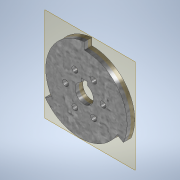
# Autodesk Inventor part: Weapon
Saved by Autodesk Inventor 2022 (Build 260153000, 153)
## iProperties
Created: 2022-08-11
Part Number: Weapon
Material: Steel
Document SubType Name: Sheet Metal
Designer: Nick
Density: 7.85 g/cm^3
Appearance: Steel Galvanized
Mass: 169.361 g
Surface Area: 86.0381 cm^2
Volume: 21.5746 cm^3
Flat Pattern Width: 6.80954 cm
Flat Pattern Length: 7.10597 cm
Flat Pattern Area: 48.3884 cm^2
Sheet Metal Rule: Default
Sheet Metal Width: 2.681 in
Sheet Metal Length: 2.798 in
Sheet Metal Area: 7.500 in^2
Author: Nick
Autodesk Inventor part; units mm, degrees
ref_plane "YZ Plane" through (0, 0, 0) normal (1, 0, 0) x (0, 1, 0)
ref_plane "XZ Plane" through (0, 0, 0) normal (0, 1, 0) x (-1, 0, 0)
ref_plane "XY Plane" through (0, 0, 0) normal (0, 0, 1) x (1, 0, 0)
sketch "Sketch1" plane through (0, 0, 0) normal (0, 0, 1) x (1, 0, 0)
  circle A0 centre (0, 0) radius 37.5 construction
  circle A1 centre (0, 0) radius 31.5
  line L0 (0, 31.5) -> (0, 37.5)
  arc A2 (0, 37.5) -> (-27.2798, -15.75) centre (3.5675, 2.0597) ccw
  line L1 (0, 0) -> (-27.2798, -15.75) construction
  circle A3 centre (0, 0) radius 7.5
  line L2 (-2.5, 10) -> (2.5, 10)
  line L3 (2.5, 10) -> (2.5, 5)
  line L4 (2.5, 5) -> (-2.5, 5)
  line L5 (-2.5, 5) -> (-2.5, 10)
  point P0 (0, 5)
  point P1 (0, 7.5)
  point P2 (2.5, 7.5)
  point P3 (2.5, 7.0711)
  point P4 (-2.5, 7.0711)
  dimension "d0" = 75
  dimension "d8" = 15
  dimension "d1" = 120
  dimension "d2" = 6
  dimension "d20" = 5
  dimension "d21" = 5
  constraints: 12 end point, 4 point on circle, 4 vertical alignment, 3 coincident, 2 centre point, 2 midpoint, 2 parallel, 1 horizontal, 1 horizontal alignment, 1 perpendicular, 1 tangent, 1 vertical, 5 other
  measures "d1" angle of L0 L1
  measures "d2" distance of L0.start L0.end
  measures "d20" distance of L2.start L2.end
  measures "d21" distance of L2.end L3.end
extrude "Extrusion1" add sketch "Sketch1" along normal blind 6.35 contours A1
extrude "Extrusion2" add sketch "Sketch1" along normal blind 6.35 contours A1 A2 L0
pattern_circular "Circular Pattern1" count 3 over 360 about axis through (0, 0, 0) along (0, 0, 1) of "Extrusion2"
ref_plane "Work Plane1" through (0, 0, 3.175) normal (0, 0, 1) x (1, 0, 0)
thicken "Thicken1" operation add thickness 0.127 both sides no extend neighbours yes toward (-0.4087164, 0.9126614, 0) faces at (-3.0654, 6.845, 4.2333) (-2.5, 8.0474, 2.1167) (-0.8333, 10, 4.2333) (2.5, 9.0237, 2.1167)
sketch "Sketch3" plane through (0, 0, 6.35) normal (0, 0, 1) x (1, 0, 0)
  circle A0 centre (0, 0) radius 15.5847
  arc A1 (-2.627, 7.1603) -> (2.627, 7.1603) centre (0, 0) ccw projected
  circle A2 centre (0, 0) radius 7.627
  arc A3 (32.476, -18.75) -> (0, 31.5) centre (0, -4.1194) ccw projected
  circle A4 centre (0, 0) radius 31.5
  point P0 (15.5847, 0)
  dimension "d26" = 15.9153
  dimension "d27" = 7.9577
  constraints: 3 coincident, 2 horizontal alignment, 1 vertical alignment, 7 other
hole "Hole2" at (15.5847, 0, 6.35) direction (0, 0, -1) diameter 5 depth 6.35
pattern_circular "Circular Pattern3" count 6 over 360 about axis through (0, 0, 0) along (0, 0, 1) of "Hole2"
equation "\"d27\" = 0.5 * d26"
equation "\"d33\" = Thickness"
equation "\"BendRadius\" = Thickness"
equation "\"BendReliefWidth\" = Thickness"
equation "\"BendReliefDepth\" = 0.5 * Thickness"
equation "\"CornerReliefSize\" = 4 * Thickness"
equation "\"MinimumRemnant\" = 2 * Thickness"
equation "\"TransitionRadius\" = BendRadius"
equation "\"JacobiRadiusSize\" = BendRadius"
equation "\"GapSize\" = Thickness"
equation "\"Thickness\" = 6.35"
body "Solid1"
